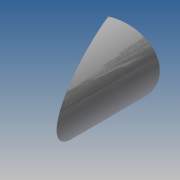
# Autodesk Inventor part: A1-19037-200-01 Trunk shell
Saved by Autodesk Inventor 2017.3 (Build 213257000, 257)
## iProperties
Created: 2019-08-22
Part Number: A1-19037-200-01 Trunk shell
Material: Steel, Mild
Document SubType Name: Sheet Metal
Designer: GVD
Density: 7.85 g/cm^3
Appearance: Steel
Project: A1-19037--CNUL Albian CST laterals
Mass: 311036 g
Surface Area: 22722.5 cm^2
Volume: 39622.4 cm^3
Description: 112 5/16" x 68 15/32" x 1 1/2" PLATE, A516 Gr.70N, ROLLED TO 37 1/4" OD
Flat Pattern Width: 124.262 cm
Flat Pattern Length: 126.909 cm
Flat Pattern Area: 15770 cm^2
Sheet Metal Rule: Default
Sheet Metal Width: 48.922 in
Sheet Metal Length: 49.964 in
Sheet Metal Area: 2444.354 in^2
Constructed By: Graeme_Van_Dongen
Project Name: CST laterals
Author: GVD
Autodesk Inventor part; units mm, degrees
ref_plane "YZ Plane" through (0, 0, 0) normal (1, 0, 0) x (0, 1, 0)
ref_plane "XZ Plane" through (0, 0, 0) normal (0, 1, 0) x (-1, 0, 0)
ref_plane "XY Plane" through (0, 0, 0) normal (0, 0, 1) x (1, 0, 0)
sketch "Sketch1" plane through (0, 0, 0) normal (0, 0, 1) x (1, 0, 0)
  circle A0 centre (0, 0) radius 409.575
  circle A1 centre (0, 0) radius 447.675
  circle A2 centre (0, 0) radius 411.1625
  dimension "d0" = 819.15
  dimension "d1" = 895.35
  dimension "d10" = 822.325
  constraints: 3 centre point, 3 coincident
  measures "d0" diameter of A0
  measures "d1" diameter of A1
  measures "d10" diameter of A2
extrude "Extrusion1" add sketch "Sketch1" along normal blind 1294.4 and the other way blind 444.4 contours A1 | A2
sketch "Sketch2" plane through (0, 0, 0) normal (0, 1, 0) x (-1, 0, 0)
  line L0 (0, 0) -> (-447.675, 1080.7831)
  line L1 (-447.675, -444.4) -> (-447.675, 1294.4) projected
  line L2 (-447.675, 1080.7831) -> (-447.675, -185.4331)
  line L3 (-447.675, -444.4) -> (-447.675, 1294.4) projected
  line L4 (0, 0) -> (-447.675, -185.4331)
  dimension "d79" = 22.5
  constraints: 6 end point, 2 point on line, 1 coincident, 1 perpendicular
  measures "d79" angle of L1 L0
extrude "Extrusion2" cut sketch "Sketch2" along normal through all both and the other way through all keep common part
ref_plane "Work Plane1" through (-288.0343, 2.1137, -447.675) normal (0.9261767, -0.3770897, 0) x (0, 0, -1)
equation "\"BendRadius\" = Thickness"
equation "\"BendReliefWidth\" = Thickness"
equation "\"BendReliefDepth\" = 0.5 * Thickness"
equation "\"CornerReliefSize\" = 4 * Thickness"
equation "\"MinimumRemnant\" = 2 * Thickness"
equation "\"TransitionRadius\" = BendRadius"
equation "\"JacobiRadiusSize\" = Thickness"
equation "\"GapSize\" = Thickness"
equation "\"Thickness\" = 38.1"
body "Solid1"
